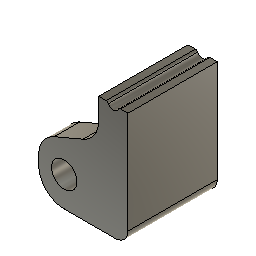
M-1Hingev3 (Autodesk Fusion 360 design; units mm, degrees)
Autodesk Fusion 360 part; units mm, degrees
sketch "Sketch1" plane through (0, 0, 0) normal (0, 1, 0) x (1, 0, 0)
  line L0 (2, 0) -> (7, 0)
  line L1 (7, 0) -> (7, -9)
  line L2 (7, -9) -> (4.7, -9)
  line L3 (4.7, -9) -> (4.7, -7.3225)
  line L4 (0, -2) -> (0, -2.6775)
  line L5 (1.2169, -4.5178) -> (3.4831, -5.4822)
  arc A0 (4.7, -7.3225) -> (3.4831, -5.4822) centre (2.7, -7.3225) ccw
  arc A1 (0, -2.6775) -> (1.2169, -4.5178) centre (2, -2.6775) ccw
  arc A2 (2, 0) -> (0, -2) centre (2, -2) ccw
  circle A3 centre (2, -2.3388) radius 1
  point P0 (4.7, -6)
  point P1 (0, -4)
  dimension "d1" = 7
  dimension "d3" = 2.3
  dimension "d4" = 3
  dimension "d5" = 4
  dimension "d6" = 2
  dimension "d7" = 2
  dimension "d8" = 2
  dimension "d10" = 2
  constraint horizontal L0
  constraint vertical L1
  constraint perpendicular L1 L2
  constraint perpendicular L2 L3
  constraint perpendicular L0 L4
  constraint coincident P0 L3
  constraint coincident P0 L5
  constraint tangent L3 A0
  constraint tangent L5 A0
  constraint coincident P1 L4
  constraint coincident P1 L5
  constraint tangent L4 A1
  constraint tangent L5 A1
  constraint coincident origin L0
  constraint coincident origin L4
  constraint tangent L0 A2
  constraint tangent L4 A2
  measures "d1" distance of origin L0.end
  measures "d3" distance of L1.end L2.end
  measures "d4" distance of L2.end P0
  measures "d5" distance of origin P1
  measures "d6" radius of A0
  measures "d7" radius of A1
  measures "d8" radius of A2
  measures "d10" diameter of A3
extrude "Extrude1" add sketch "Sketch1" along normal blind 7
sketch "Sketch2" plane through (0, 0, 9) normal (0, 0, 1) x (-1, 0, 0)
  line L0 (-4.7, 0) -> (-7, 0)
  line L1 (-7, 0) -> (-7, -7)
  line L2 (-7, -7) -> (-4.7, -7)
  line L3 (-4.7, -7) -> (-4.7, 0)
  line L4 (-4.7, -7) -> (0, -7)
  line L5 (0, -7) -> (0, -5)
  line L6 (0, -5) -> (-4.7, -5)
  line L7 (-4.7, -5) -> (-4.7, -7)
  line L8 (-4.7, 0) -> (0, 0)
  line L9 (0, 0) -> (0, -2)
  line L10 (0, -2) -> (-4.7, -2)
  line L11 (-4.7, -2) -> (-4.7, 0)
  line L12 (0, -5) -> (-4.7, -5)
  line L13 (-4.7, -5) -> (-4.7, -2)
  line L14 (-4.7, -2) -> (0, -2)
  line L15 (0, -2) -> (0, -5)
  constraint horizontal L4
  constraint vertical L5
  constraint horizontal L6
  constraint vertical L7
  constraint coincident L2.end L3.start
  constraint horizontal L8
  constraint vertical L9
  constraint horizontal L10
  constraint vertical L11
  constraint coincident L0.start L3.end
  constraint horizontal L12
  constraint vertical L13
  constraint horizontal L14
  constraint vertical L15
extrude "Extrude2" cut sketch "Sketch2" against normal blind 10 contours L3 L6 L10 L12 L13 L14 L15
sketch "Sketch3" plane through (4.7, 0, 0) normal (-1, 0, 0) x (0, -1, 0)
  line L0 (0, 9) -> (-7, 9)
  line L1 (-7, 9) -> (-7, 7.3225)
  line L2 (-7, 7.3225) -> (-5, 7.3225)
  line L3 (-5, 7.3225) -> (-5, 0)
  line L4 (-5, 0) -> (-2, 0)
  line L5 (-2, 0) -> (-2, 7.3225)
  line L6 (-2, 7.3225) -> (0, 7.3225)
  line L7 (0, 7.3225) -> (0, 9)
  line L8 (-3.75, 7) -> (-3.25, 7)
  line L9 (-2.5, 6.25) -> (-2.5, 1.25)
  line L10 (-3.25, 0.5) -> (-3.75, 0.5)
  line L11 (-4.5, 1.25) -> (-4.5, 6.25)
  arc A0 (-3.75, 7) -> (-4.5, 6.25) centre (-3.75, 6.25) ccw
  arc A1 (-2.5, 6.25) -> (-3.25, 7) centre (-3.25, 6.25) ccw
  arc A2 (-4.5, 1.25) -> (-3.75, 0.5) centre (-3.75, 1.25) ccw
  arc A3 (-3.25, 0.5) -> (-2.5, 1.25) centre (-3.25, 1.25) ccw
  dimension "d15" = 0.75
  constraint horizontal L8
  constraint vertical L9
  constraint horizontal L10
  constraint vertical L11
  constraint tangent L8 A0
  constraint tangent L11 A0
  constraint tangent L8 A1
  constraint tangent L9 A1
  constraint equal A0 A1
  constraint tangent L10 A2
  constraint tangent L11 A2
  constraint equal A0 A2
  constraint tangent L9 A3
  constraint tangent L10 A3
  constraint equal A0 A3
  measures "d15" radius of A0
extrude "Extrude3" cut sketch "Sketch3" against normal blind 0.2 contours L8 L9 L10 L11 A0 A1 A2 A3
fillet "Fillet1" radius 0.1 8 edges at (4.9, 3.5, 7) (4.9, 2.7197, 6.7803) (4.9, 2.5, 3.75) (4.9, 2.7197, 0.7197) (4.9, 3.5, 0.5) (4.9, 4.2803, 0.7197) (4.9, 4.5, 3.75) (4.9, 4.2803, 6.7803)
sketch "Sketch4" plane through (0, 0, 0) normal (0, -1, 0) x (1, 0, 0)
  circle A0 centre (2, 2.3388) radius 1
  line L0 (2, 0) -> (7, 0)
  line L1 (7, 0) -> (7, 9)
  line L2 (7, 9) -> (4.7, 9)
  line L3 (4.7, 9) -> (4.7, 7.3225)
  arc A1 (3.4831, 5.4822) -> (4.7, 7.3225) centre (2.7, 7.3225) ccw
  line L4 (3.4831, 5.4822) -> (1.2169, 4.5178)
  arc A2 (1.2169, 4.5178) -> (0, 2.6775) centre (2, 2.6775) ccw
  line L5 (0, 2.6775) -> (0, 2)
  arc A3 (0, 2) -> (2, 0) centre (2, 2) ccw
  line L6 (4.7, 9) -> (5.43, 9)
  line L7 (7, 9) -> (6.27, 9)
  arc A4 (5.43, 9) -> (6.27, 9) centre (5.85, 9.066) ccw
  line L8 (5.43, 9) -> (6.27, 9)
  dimension "d20" = 0.73
  dimension "d21" = 0.73
  constraint coincident L2.end L3.start
  constraint perpendicular L3 L6
  constraint coincident L1.end L2.start
  constraint coincident L2 L7.end
  measures "d20" distance of L2.end L6.end
  measures "d21" distance of L1.end L7.end
extrude "Extrude4" cut sketch "Sketch4" against normal blind 7 contours L2 A4 L8
fillet "Fillet2" radius 0.2 2 edges at (5.43, 3.5, 9) (6.27, 3.5, 9)
fillet "Fillet4" radius 1 1 edges at (7, 3.5, 0)
sketch "Sketch5" plane through (0, 0, 0) normal (0, 0, -1) x (1, 0, 0)
  line L0 (6, -7) -> (6, 0)
  line L1 (6, 0) -> (2, 0)
  line L2 (2, 0) -> (2, -2)
  line L3 (2, -2) -> (4.7, -2)
  line L4 (4.7, -2) -> (4.7, -5)
  line L5 (4.7, -5) -> (2, -5)
  line L6 (2, -5) -> (2, -7)
  line L7 (2, -7) -> (6, -7)
  line L8 (7, 0) -> (6.24, 0)
  line L9 (6.24, 0) -> (5.24, 0)
  line L10 (5.24, 0) -> (5.24, -6.5)
  line L11 (6.24, -6.5) -> (6.24, 0)
  line L12 (5.24, 0) -> (5.24, -0.5)
  line L13 (5.24, -0.5) -> (6.24, -0.5)
  line L14 (5.24, -6.5) -> (6.24, -6.5)
  dimension "d30" = 0.76
  dimension "d31" = 1
  dimension "d33" = 0.5
  constraint perpendicular L0 L8
  constraint horizontal L9
  constraint vertical L10
  constraint vertical L11
  constraint perpendicular L9 L12
  constraint coincident L11 L13.end
  constraint perpendicular L11 L13
  constraint perpendicular L11 L14
  measures "d30" distance of L8.start L8.end
  measures "d31" distance of L8.end L9.end
  measures "d33" distance of L9.end L12.end
extrude "Extrude5" cut sketch "Sketch5" against normal blind 7 contours L0 L10 L13 L14 | L0 L11 L13 L14
fillet "Fillet5" radius 0.1 8 edges at (4.7, 3.5, 7) (4.7, 2.7197, 6.7803) (4.7, 2.5, 3.75) (4.7, 2.7197, 0.7197) (4.7, 3.5, 0.5) (4.7, 4.2803, 0.7197) (4.7, 4.5, 3.75) (4.7, 4.2803, 6.7803)
